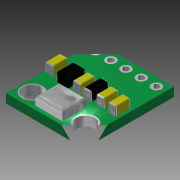
# Autodesk Inventor part: BMP180_SHEELD_13x15
Saved by Autodesk Inventor 2014 SP1 (Build 180222100, 222)
## iProperties
Created: 2015-09-18
Part Number: BMP180_SHEELD_13x15
Material: Типовые
Document SubType Name: Modeling
Designer: Oleg
Density: 1 g/cm^3
Appearance: По умолчанию
Author: Oleg
Autodesk Inventor part; units mm, degrees
ref_plane "YZ Plane" through (0, 0, 0) normal (1, 0, 0) x (0, 1, 0)
ref_plane "XZ Plane" through (0, 0, 0) normal (0, 1, 0) x (-1, 0, 0)
ref_plane "XY Plane" through (0, 0, 0) normal (0, 0, 1) x (1, 0, 0)
sketch "Эскиз1" plane through (0, 0, 0) normal (0, 0, 1) x (1, 0, 0)
  line L0 (13.1, -15) -> (0, -15)
  line L1 (0, -15) -> (0, 0)
  line L2 (0, 0) -> (13.1, 0)
  line L3 (13.1, 0) -> (13.1, -15)
  circle A0 centre (2.1, -12.7) radius 1.5
  circle A1 centre (11, -12.7) radius 1.5
  circle A2 centre (1.5, -1.5) radius 0.5
  circle A3 centre (4.04, -1.5) radius 0.5
  circle A4 centre (6.58, -1.5) radius 0.5
  circle A5 centre (9.12, -1.5) radius 0.5
  circle A6 centre (11.66, -1.5) radius 0.5
  dimension "d0" = 13.1
  dimension "d1" = 15
  dimension "d2" = 3
  dimension "d3" = 2.3
  dimension "d4" = 2.3
  dimension "d5" = 2.1
  dimension "d6" = 2.1
  dimension "d7" = 1
  dimension "d8" = 1.5
  dimension "d9" = 1.5
  dimension "d10" = 2.54
  dimension "d11" = 1.5
  dimension "d12" = 1.5
  dimension "d13" = 1.5
  dimension "d14" = 1.5
  dimension "d15" = 2.54
  dimension "d16" = 2.54
  dimension "d17" = 2.54
  constraints: 8 end point, 7 centre point, 5 equal radius, 2 parallel, 1 coincident, 1 horizontal, 1 perpendicular
  measures "d0" distance of L1.end L2.end
  measures "d1" distance of L2.end L0.start
  measures "d2" diameter of A0
  measures "d3" distance from line of L0 A0.centre
  measures "d4" distance from line of L0 A1.centre
  measures "d5" distance from line of L3 A1.centre
  measures "d6" distance from line of L1 A0.centre
  measures "d7" diameter of A2
  measures "d8" distance from line of L2 A2.centre
  measures "d9" distance from line of L1 A2.centre
  measures "d10" distance of A3.centre A2.centre
  measures "d11" distance from line of L2 A3.centre
  measures "d12" distance from line of L2 A4.centre
  measures "d13" distance from line of L2 A5.centre
  measures "d14" distance from line of L2 A6.centre
  measures "d15" distance of A3.centre A4.centre
  measures "d16" distance of A4.centre A5.centre
  measures "d17" distance of A5.centre A6.centre
extrude "Выдавливание1" add sketch "Эскиз1" along normal blind 1.5
sketch "Эскиз2" plane through (0, 0, 1.5) normal (0, 0, 1) x (1, 0, 0)
  line L0 (0, -15) -> (13.1, -15) projected
  line L1 (0, 0) -> (0, -15) projected
  line L2 (8.77, -14.3602) -> (4.27, -14.3602)
  line L3 (4.27, -14.3602) -> (4.27, -10.3602)
  line L4 (4.27, -10.3602) -> (8.77, -10.3602)
  line L5 (8.77, -10.3602) -> (8.77, -14.3602)
  line L6 (12.5994, -9.2437) -> (11.2994, -9.2437)
  line L7 (11.2994, -9.2437) -> (11.2994, -6.7437)
  line L8 (11.2994, -6.7437) -> (12.5994, -6.7437)
  line L9 (12.5994, -6.7437) -> (12.5994, -9.2437)
  line L10 (10.4582, -9.1058) -> (9.1582, -9.1058)
  line L11 (9.1582, -9.1058) -> (9.1582, -6.6058)
  line L12 (9.1582, -6.6058) -> (10.4582, -6.6058)
  line L13 (10.4582, -6.6058) -> (10.4582, -9.1058)
  line L14 (8.4172, -9.2437) -> (7.1172, -9.2437)
  line L15 (7.1172, -9.2437) -> (7.1172, -6.1922)
  line L16 (7.1172, -6.1922) -> (8.4172, -6.1922)
  line L17 (8.4172, -6.1922) -> (8.4172, -9.2437)
  line L18 (6.4887, -9.0485) -> (5.1887, -9.0485)
  line L19 (5.1887, -9.0485) -> (5.1887, -6.5485)
  line L20 (5.1887, -6.5485) -> (6.4887, -6.5485)
  line L21 (6.4887, -6.5485) -> (6.4887, -9.0485)
  line L22 (4.5807, -9.129) -> (2.5807, -9.129)
  line L23 (2.5807, -9.129) -> (2.5807, -6.329)
  line L24 (2.5807, -6.329) -> (4.5807, -6.329)
  line L25 (4.5807, -6.329) -> (4.5807, -9.129)
  line L26 (1.4973, -8.6757) -> (0.1973, -8.6757)
  line L27 (0.1973, -8.6757) -> (0.1973, -6.1757)
  line L28 (0.1973, -6.1757) -> (1.4973, -6.1757)
  line L29 (1.4973, -6.1757) -> (1.4973, -8.6757)
  dimension "d21" = 0.6398
  dimension "d22" = 4.27
  dimension "d23" = 4
  dimension "d24" = 4.5
  dimension "d25" = 1.3
  dimension "d26" = 2.5
  dimension "d27" = 2.8
  dimension "d28" = 2
  constraints: 56 end point, 14 parallel, 7 equal length, 7 horizontal, 7 perpendicular
  measures "d21" distance between parallel lines of L0 L2
  measures "d22" distance between parallel lines of L1 L3
  measures "d23" distance of L4.end L2.start
  measures "d24" distance of L3.end L4.end
  measures "d25" distance of L6.start L6.end
  measures "d26" distance between parallel lines of L6 L8
  measures "d27" distance between parallel lines of L24 L22
  measures "d28" distance of L22.start L22.end
extrude "Выдавливание2" add sketch "Эскиз2" along normal blind 1.5
sketch "Эскиз3" plane through (0, 0, 1.5) normal (0, 0, 1) x (1, 0, 0)
  circle A0 centre (11.66, -1.5) radius 0.5 projected
  circle A1 centre (9.12, -1.5) radius 0.5 projected
  circle A2 centre (6.58, -1.5) radius 0.5 projected
  circle A3 centre (4.04, -1.5) radius 0.5 projected
  circle A4 centre (1.5, -1.5) radius 0.5 projected
  line L0 (13.1, 0) -> (0, 0) projected
  circle A5 centre (1.5, -1.5) radius 0.8
  circle A6 centre (4.04, -1.5) radius 0.8
  circle A7 centre (6.58, -1.5) radius 0.8
  circle A8 centre (9.12, -1.5) radius 0.8
  circle A9 centre (11.66, -1.5) radius 0.8
  dimension "d38" = 1.6
  dimension "d41" = 2.54
  constraints: 5 centre point, 1 coincident, 1 horizontal, 8 other
  measures "d38" diameter of A5
  measures "d41" distance of A5.centre A6.centre
extrude "Выдавливание3" add sketch "Эскиз3" along normal blind 0.05
fillet "Сопряжение1" radius 0.5 4 edges at (8.77, -12.3602, 3) (6.52, -10.3602, 3) (4.27, -12.3602, 3) (6.52, -14.3602, 3)
fillet "Сопряжение2" radius 0.2 32 edges at (12.5994, -7.9937, 3) (11.2994, -7.9937, 3) (11.9494, -6.7437, 3) (12.5994, -6.7437, 2.25) (11.2994, -6.7437, 2.25) (11.9494, -9.2437, 3) (11.2994, -9.2437, 2.25) (12.5994, -9.2437, 2.25) (10.4582, -9.1058, 2.25) (9.8082, -9.1058, 3) (9.1582, -9.1058, 2.25) (9.1582, -7.8558, 3) (10.4582, -7.8558, 3) (9.8082, -6.6058, 3) (10.4582, -6.6058, 2.25) (9.1582, -6.6058, 2.25) (0.8473, -8.6757, 3) (1.4973, -8.6757, 2.25) (1.4973, -7.4257, 3) (0.1973, -7.4257, 3) (0.8473, -6.1757, 3) (1.4973, -6.1757, 2.25) (0.1973, -6.1757, 2.25) (0.1973, -8.6757, 2.25) (5.8387, -6.5485, 3) (6.4887, -7.7985, 3) (5.1887, -7.7985, 3) (5.8387, -9.0485, 3) (6.4887, -6.5485, 2.25) (5.1887, -6.5485, 2.25) (6.4887, -9.0485, 2.25) (5.1887, -9.0485, 2.25)
fillet "Сопряжение3" radius 0.2 16 edges at (8.4172, -7.718, 3) (7.1172, -7.718, 3) (7.7672, -6.1922, 3) (8.4172, -6.1922, 2.25) (7.1172, -6.1922, 2.25) (8.4172, -9.2437, 2.25) (7.1172, -9.2437, 2.25) (7.7672, -9.2437, 3) (4.5807, -7.729, 3) (3.5807, -6.329, 3) (4.5807, -6.329, 2.25) (2.5807, -6.329, 2.25) (2.5807, -7.729, 3) (3.5807, -9.129, 3) (2.5807, -9.129, 2.25) (4.5807, -9.129, 2.25)
sketch "Эскиз4" plane through (0, 0, 0) normal (0, 0, -1) x (-1, 0, 0)
  circle A0 centre (-11.66, -1.5) radius 0.5 projected
  circle A1 centre (-9.12, -1.5) radius 0.5 projected
  circle A2 centre (-6.58, -1.5) radius 0.5 projected
  circle A3 centre (-4.04, -1.5) radius 0.5 projected
  circle A4 centre (-1.5, -1.5) radius 0.5 projected
  line L0 (0, 0) -> (-13.1, 0) projected
  circle A5 centre (-11.66, -1.5) radius 0.8
  circle A6 centre (-9.12, -1.5) radius 0.8
  circle A7 centre (-6.58, -1.5) radius 0.8
  circle A8 centre (-4.04, -1.5) radius 0.8
  circle A9 centre (-1.5, -1.5) radius 0.8
  dimension "d51" = 1.6
  dimension "d54" = 2.54
  constraints: 5 centre point, 1 coincident, 1 horizontal, 8 other
  measures "d51" diameter of A5
  measures "d54" distance of A5.centre A6.centre
extrude "Выдавливание4" add sketch "Эскиз4" along normal blind 0.05
sketch "Эскиз6" plane through (0, 0, 1.5) normal (0, 0, 1) x (1, 0, 0)
  circle A0 centre (11, -12.7) radius 1.5 projected
  circle A1 centre (2.1, -12.7) radius 1.5 projected
  circle A2 centre (2.1, -12.7) radius 1.75
  circle A3 centre (11, -12.7) radius 1.75
  dimension "d71" = 3.5
  constraints: 2 centre point, 2 coincident, 1 equal radius
  measures "d71" diameter of A3
extrude "Выдавливание6" add sketch "Эскиз6" along normal blind 0.05
sketch "Эскиз7" plane through (0, 0, 0) normal (0, 0, -1) x (-1, 0, 0)
  circle A0 centre (-11, -12.7) radius 1.5 projected
  circle A1 centre (-2.1, -12.7) radius 1.5 projected
  circle A2 centre (-11, -12.7) radius 1.75 projected
  circle A3 centre (-2.1, -12.7) radius 1.75 projected
extrude "Выдавливание7" add sketch "Эскиз7" along normal blind 0.05
sketch "Эскиз8" plane through (0, 0, 1.5) normal (0, 0, 1) x (1, 0, 0)
  line L0 (2.5807, -8.929) -> (2.5807, -6.529) projected
  line L1 (4.5807, -6.529) -> (4.5807, -8.929) projected
  line L2 (4.3807, -9.129) -> (2.7807, -9.129) projected
  line L3 (2.5807, -8.8692) -> (2.1807, -8.8692)
  line L4 (2.1807, -8.8692) -> (2.1807, -8.3692)
  line L5 (2.1807, -8.3692) -> (2.5807, -8.3692)
  line L6 (2.5807, -8.3692) -> (2.5807, -8.8692)
  line L7 (2.5807, -7.9692) -> (2.1807, -7.9692)
  line L8 (2.1807, -7.9692) -> (2.1807, -7.4692)
  line L9 (2.1807, -7.4692) -> (2.5807, -7.4692)
  line L10 (2.5807, -7.4692) -> (2.5807, -7.9692)
  line L11 (2.5807, -7.0363) -> (2.1807, -7.0363)
  line L12 (2.1807, -7.0363) -> (2.1807, -6.5363)
  line L13 (2.1807, -6.5363) -> (2.5807, -6.5363)
  line L14 (2.5807, -6.5363) -> (2.5807, -7.0363)
  line L15 (4.5807, -8.429) -> (4.9807, -8.429)
  line L16 (4.9807, -8.429) -> (4.9807, -7.929)
  line L17 (4.9807, -7.929) -> (4.5807, -7.929)
  line L18 (4.5807, -7.929) -> (4.5807, -8.429)
  line L19 (4.5807, -7.529) -> (4.9807, -7.529)
  line L20 (4.9807, -7.529) -> (4.9807, -7.029)
  line L21 (4.9807, -7.029) -> (4.5807, -7.029)
  line L22 (4.5807, -7.029) -> (4.5807, -7.529)
  dimension "d76" = 0.5
  dimension "d77" = 0.4
  dimension "d78" = 0.4
  dimension "d79" = 0.5
  dimension "d80" = 0.7
  dimension "d81" = 0.4
  dimension "d82" = 0.4
  constraints: 40 end point, 10 parallel, 6 equal length, 5 horizontal, 5 perpendicular, 5 point on line
  measures "d76" distance of L3.end L4.end
  measures "d77" distance of L4.end L5.end
  measures "d78" distance of L19.start L19.end
  measures "d79" distance of L15.end L16.end
  measures "d80" distance between parallel lines of L2 L15
  measures "d81" distance between parallel lines of L7 L5
  measures "d82" distance between parallel lines of L19 L17
extrude "Выдавливание8" add sketch "Эскиз8" along normal blind 0.2
fillet "Сопряжение4" radius 0.05 25 edges at (2.1807, -6.7863, 1.7) (2.3807, -6.5363, 1.7) (2.3807, -7.0363, 1.7) (2.1807, -7.0363, 1.6) (2.1807, -6.5363, 1.6) (2.3807, -7.4692, 1.7) (2.1807, -7.7192, 1.7) (2.1807, -7.4692, 1.6) (2.3807, -7.9692, 1.7) (2.1807, -7.9692, 1.6) (2.3807, -8.3692, 1.7) (2.1807, -8.3692, 1.6) (2.1807, -8.6192, 1.7) (2.3807, -8.8692, 1.7) (2.1807, -8.8692, 1.6) (4.7807, -7.029, 1.7) (4.9807, -7.279, 1.7) (4.9807, -7.029, 1.6) (4.9807, -7.529, 1.6) (4.7807, -7.529, 1.7) (4.7807, -8.429, 1.7) (4.9807, -8.429, 1.6) (4.9807, -8.179, 1.7) (4.9807, -7.929, 1.6) (4.7807, -7.929, 1.7)
